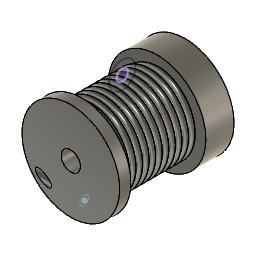
hoist (Autodesk Fusion 360 archive; units mm, degrees)
design "rope-drum"
Autodesk Fusion 360 part; units mm, degrees
note: some values were not read from the file. Chosen so that the rebuilt part matches the saved one: the hand of a thread or coil; which pieces of a blend or face edit are solid.
sketch "Sketch1" plane through (0, 0, 0) normal (1, 0, 0) x (0, 1, 0) in component "pulley"
  line L0 (0, 0) -> (-30.5, 0)
  line L1 (-30.5, 0) -> (-30.5, 13)
  line L2 (-27.5, 10.5) -> (-7.5, 10.5)
  line L3 (0, 0) -> (0, 13)
  line L4 (0, 2.55) -> (-30.5, 2.55)
  line L5 (-17.5, 10.5) -> (-17.5, 0) construction
  line L6 (0, 13) -> (-7.5, 13)
  line L7 (-7.5, 13) -> (-7.5, 10.5)
  line L8 (-27.5, 10.5) -> (-27.5, 13)
  line L9 (-27.5, 13) -> (-30.5, 13)
  line L10 (-7.5, 10.5) -> (-7.5, 0)
  line L11 (-27.5, 10.5) -> (-27.5, 0)
  dimension "d41_1" = 2.55
  dimension "d1" = 10.5
  dimension "d4" = 7.5
  dimension "d6" = 3
  dimension "d7" = 20
  dimension "d8" = 2.5
  constraint coincident L0.start L3.start
  constraint horizontal L0
  constraint perpendicular L0 L1
  constraint parallel L0 L2
  constraint perpendicular L0 L3
  constraint coincident L3 L4.start
  constraint coincident L1 L4.end
  constraint perpendicular L1 L4
  constraint midpoint L2 L5.start
  constraint vertical L5
  constraint perpendicular L3 L6
  constraint perpendicular L2 L7
  constraint perpendicular L2 L8
  constraint perpendicular L1 L9
  constraint collinear L6 L9
  constraint coincident L0 L10.end
  constraint perpendicular L0 L10
  constraint coincident L0 L11.end
  constraint perpendicular L0 L11
  measures "d41_1" distance of L0 L4
  measures "d1" distance of L0 L2
  measures "d4" distance of L3.end L6.end
  measures "d6" distance of L1.end L8.end
  measures "d7" distance of L2.start L2.end
  measures "d8" distance of L2.start L8.end
revolve "Revolve1" add sketch "Sketch1" angle 360 about axis through (0, 0, 0) along (0, -1, 0) contours L2 L4 L10 L11 makes body 1
coil "CoilPrimitive1" cut diameter 21.5 section circle size 1.75 on centre turns 16 pitch 1.75063 left hand placed x (1, 0, 0) y (0, 0, 1) z (0, -1, 0) at (0, 0, 0) bodies 1
revolve "Revolve1'" add sketch "Sketch1" angle 360 about axis through (0, 0, 0) along (0, -1, 0) separate body contours L3 L4 L6 L7 L10 | L1 L4 L8 L9 L11 makes body 2 at (0.648, -5, 12.9838) makes body 3 at (0.6458, -30.5, 9.4683) in component "pulley"
sketch "Sketch3" plane through (0, 0, 0) normal (0, 1, 0) x (-1, 0, 0) in component "pulley"
  circle A0 centre (0, 0) radius 2.55
  line L0 (3.15, 3.1) -> (5.56, 3.1)
  line L1 (5.56, 3.1) -> (5.56, -3.1)
  line L2 (5.56, -3.1) -> (3.15, -3.1)
  line L3 (3.15, -3.1) -> (3.15, 3.1)
  line L4 (0, 0) -> (3.15, 0) construction
  circle A1 centre (0, 0) radius 13
  circle A2 centre (0, 0) radius 8.5
  circle A3 centre (0, 0) radius 8.5
  dimension "d152_1" = 2.41
  dimension "d153_1" = 6.2
  dimension "d154_1" = 0.6
  constraint horizontal L0
  constraint vertical L1
  constraint horizontal L2
  constraint vertical L3
  constraint coincident A0.centre L4.start
  constraint midpoint L3 L4.end
  constraint horizontal L4
  measures "d152_1" distance of L0.start L0.end
  measures "d153_1" distance of L0.end L1.end
  measures "d154_1" distance of A0 L3
extrude "Extrude1" cut sketch "Sketch3" against normal blind 6.5 contours L0 L1 L2 L3 bodies 2 in component "pulley"
sketch "Sketch4" plane through (-5.56, 0, 0) normal (1, 0, 0) x (0, 1, 0) in component "pulley"
  line L0 (0, -3.1) -> (0, 3.1)
  line L1 (0, 3.1) -> (-6.5, 3.1)
  line L2 (-6.5, 3.1) -> (-6.5, -3.1)
  line L3 (-6.5, -3.1) -> (0, -3.1)
  circle A0 centre (-3.78, 0) radius 1.5
  line L4 (-6.5, 0) -> (0, 0) construction
  line L5 (-3.78, 3.1408) -> (-6.5, 1.5704)
  line L6 (-6.5, 1.5704) -> (-6.5, -1.5704)
  line L7 (-6.5, -1.5704) -> (-3.78, -3.1408)
  line L8 (-3.78, -3.1408) -> (-1.06, -1.5704)
  line L9 (-1.06, -1.5704) -> (-1.06, 1.5704)
  line L10 (-1.06, 1.5704) -> (-3.78, 3.1408)
  point P0 (-3.78, 0)
  point P1 (-3.78, 0)
  dimension "d149_1" = 3
  dimension "d151_1" = 2.72
  constraint coincident P1 P0
  constraint midpoint L2 L4.start
  constraint coincident L4.end origin
  constraint coincident P1 L4
  constraint collinear L2 L6
  measures "d149_1" diameter of A0
  measures "d151_1" distance of P1 L10
extrude "Extrude2" cut sketch "Sketch4" against normal through all and the other way up to surface contours A0 second end surface at (0.1271, -2.5, 2.5468) on bodies 2 bodies 2 in component "pulley"
combine "Combine2" operation add target body 3 tool bodies 2 1 in component "pulley"
sketch "Sketch10" plane through (0, 0, 0) normal (1, 0, 0) x (0, 1, 0)
  circle A0 centre (-26.862, -10.9614) radius 1.125
  dimension "d25" = 2.25
  measures "d25" diameter of A0
extrude "Extrude1'" add sketch "Sketch10" against normal blind 12 separate body makes body 4
move_face "MoveFace1" to x (0.760804, 0.451444, -0.466235) y (-0.637527, 0.654266, -0.406811) z (0.121389, 0.606741, 0.785576) at (-19.7681, -4.3049, -11.8644) 1 faces at (-8, -26.5573, -9.8784) on bodies 4
combine "Combine3" operation cut target body 3 tool bodies 4 in component "pulley"
ref_plane "WorkPlane1" through (-13, -3.0209, 0) normal (-1, 0, 0) x (0, 0, -1)
sketch "Sketch13" plane through (-13, 0, 0) normal (-1, 0, 0) x (0, -1, 0)
  spline S0 degree 3 poles (3.78, 1.5) (3.9685, 1.5) (4.1695, 1.4623) (4.539, 1.3092) (4.7076, 1.1937) (4.9737, 0.9276) (5.0892, 0.759) (5.2423, 0.3895) (5.28, 0.1885) (5.28, -0.1885) (5.2423, -0.3895) (5.0892, -0.759) (4.9737, -0.9276) (4.7076, -1.1937) (4.539, -1.3092) (4.1695, -1.4623) (3.9685, -1.5) (3.5915, -1.5) (3.3905, -1.4623) (3.021, -1.3092) (2.8524, -1.1937) (2.5863, -0.9276) (2.4708, -0.759) (2.3177, -0.3895) (2.28, -0.1885) (2.28, 0.1885) (2.3177, 0.3895) (2.4708, 0.759) (2.5863, 0.9276) (2.8524, 1.1937) (3.021, 1.3092) (3.3905, 1.4623) (3.5915, 1.5) (3.78, 1.5) knots 0 0 0 0 0.056557 0.056557 0.113115 0.113115 0.169671 0.169671 0.226228 0.226228 0.282785 0.282785 0.339342 0.339342 0.3959 0.3959 0.452457 0.452457 0.509014 0.509014 0.565571 0.565571 0.622128 0.622128 0.678685 0.678685 0.735242 0.735242 0.791799 0.791799 0.848356 0.848356 0.904914 0.904914 0.904914 0.904914
  circle A0 centre (3.78, 0) radius 1.5
  spline S1 degree 3 poles (3.78, 1.5) (3.9685, 1.5) (4.1695, 1.4623) (4.539, 1.3092) (4.7076, 1.1937) (4.9737, 0.9276) (5.0892, 0.759) (5.2423, 0.3895) (5.28, 0.1885) (5.28, -0.1885) (5.2423, -0.3895) (5.0892, -0.759) (4.9737, -0.9276) (4.7076, -1.1937) (4.539, -1.3092) (4.1695, -1.4623) (3.9685, -1.5) (3.5915, -1.5) (3.3905, -1.4623) (3.021, -1.3092) (2.8524, -1.1937) (2.5863, -0.9276) (2.4708, -0.759) (2.3177, -0.3895) (2.28, -0.1885) (2.28, 0.1885) (2.3177, 0.3895) (2.4708, 0.759) (2.5863, 0.9276) (2.8524, 1.1937) (3.021, 1.3092) (3.3905, 1.4623) (3.5915, 1.5) (3.78, 1.5) knots 0 0 0 0 0.056557 0.056557 0.113115 0.113115 0.169671 0.169671 0.226228 0.226228 0.282785 0.282785 0.339342 0.339342 0.3959 0.3959 0.452457 0.452457 0.509014 0.509014 0.565571 0.565571 0.622128 0.622128 0.678685 0.678685 0.735242 0.735242 0.791799 0.791799 0.848356 0.848356 0.904914 0.904914 0.904914 0.904914
  circle A1 centre (3.78, 0) radius 3.5
  dimension "d29" = 7
  constraint concentric A0 A1
  measures "d29" diameter of A1
extrude "Extrude7" cut sketch "Sketch13" against normal blind 3 bodies 3 in component "pulley"
component "pulley" placed x (1, 0, 0) y (0, 1, 0) z (0, 0, 1) at (0, 0, 0)
equation "d151_1 = ( 5.44 / 2 ) * 1 mm"
equation "d1 = ( 21 / 2 ) * 1 mm"
equation "d4 = 5.5 mm + 2 mm"
